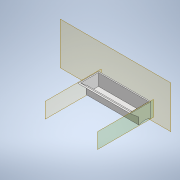
# Autodesk Inventor part: sump
Saved by Autodesk Inventor 2022 (Build 260153000, 153)
## iProperties
Created: 2022-02-25
Part Number: sump
Material: Generic
Document SubType Name: Modeling
Designer: efred
Density: 1 g/cm^3
Appearance: Default
Author: efred
Autodesk Inventor part; units mm, degrees
ref_plane "YZ Plane" through (0, 0, 0) normal (1, 0, 0) x (0, 1, 0)
ref_plane "XZ Plane" through (0, 0, 0) normal (0, 1, 0) x (-1, 0, 0)
ref_plane "XY Plane" through (0, 0, 0) normal (0, 0, 1) x (1, 0, 0)
ref_plane "Work Plane1" through (0, 0, 0) normal (0, 0, 1) x (1, 0, 0)
ref_plane "Work Plane2" through (157.5, -135.5375, 119.9) normal (1, 0, 0) x (0, 0, -1)
ref_plane "Work Plane3" through (404.675, -135.5375, 119.9) normal (-1, 0, 0) x (0, 0, 1)
sketch "Sketch2" plane through (404.675, -135.5375, 119.9) normal (-1, 0, 0) x (0, 0, 1)
  line L0 (-120, -33.125) -> (-120, 33.125) projected
  line L1 (120, -33.125) -> (-120, -33.125) projected
  line L2 (120, 33.125) -> (120, -33.125) projected
  line L3 (-120, 33.125) -> (120, 33.125) projected
  circle A0 centre (7, 26.125) radius 1.95 projected
  circle A1 centre (113, -26.875) radius 1.95 projected
  circle A2 centre (113, 12.125) radius 1.95 projected
  circle A3 centre (99, 26.125) radius 1.95 projected
  circle A4 centre (-55, -26.875) radius 1.95 projected
  line L4 (0.75, 33.125) -> (-62, -20.125) projected
  line L5 (-50.0649, 0.1287) -> (-21.3323, 24.6904) projected
  line L6 (-11.7313, 32.1577) -> (-59.0108, -8.2587) projected
  line L7 (-62, -22.3139) -> (-62, -29.97) projected
  line L8 (-119.9, -33.125) -> (-62.2, -33.125)
  line L9 (-62.2, -33.125) -> (-62.2, 33.125)
  line L10 (-62.2, 33.125) -> (-119.9, 33.125)
  line L11 (-119.9, 33.125) -> (-119.9, -33.125)
  line L12 (-62.2, 33.125) -> (-22.5461, 33.125)
  line L13 (-22.5461, 33.125) -> (-62.2, -0.7727)
  line L14 (-50.1997, 8.8278) -> (-29.9045, 26.1769) projected
  point P0 (-119.9, 135.5375)
  point P1 (-119.9, 33.125)
  point P2 (-119.9, -33.125)
  point P3 (-62.2, -33.125)
  dimension "d2" = 0.1
  dimension "d3" = 0.2
  dimension "d16" = 0.5
  constraints: 12 end point, 3 parallel, 3 point on line, 1 collinear, 1 horizontal, 1 perpendicular
  measures "d2" distance between parallel lines of L0 L11
  measures "d3" distance between parallel lines of L7 L9
  measures "d16" distance between parallel lines of L14 L13
extrude "Extrusion1" add sketch "Sketch2" along normal up to surface (247.175 mm away) contours L11 L3 L9 L1 | L3 L13 L9
shell "Shell1" thickness 5 removed faces 1 at (322.2833, -102.4125, 64.9026)
sketch "Sketch3" plane through (404.675, -135.5375, 119.9) normal (1, 0, 0) x (0, 0, -1)
  line L0 (114.9, -28.125) -> (67.2, -28.125) projected
  line L1 (67.2, -28.125) -> (67.2, 1.531) projected
  line L2 (115, 28.125) -> (115, -28.125) projected
  line L3 (67.2, -23.125) -> (115, -23.125)
  line L4 (115, -23.125) -> (115, -28.125)
  line L5 (115, -28.125) -> (67.2, -28.125)
  line L6 (67.2, -28.125) -> (67.2, -23.125)
  point P0 (119.9, 135.5375)
  point P1 (115, -23.125)
  dimension "d8" = 5
  constraints: 8 end point, 2 parallel, 1 horizontal, 1 perpendicular, 1 point on line
  measures "d8" distance between parallel lines of L0 L3
extrude "Extrusion2" add sketch "Sketch3" against normal up to surface (242.175 mm away)
sketch "Sketch4" plane through (404.675, -135.5375, 119.9) normal (1, 0, 0) x (0, 0, -1)
  line L0 (119.9, -33.125) -> (62.2, -33.125) projected
  arc A0 (114.9, -33.125) -> (67.2, -33.125) centre (91.05, -87.5073) ccw
  point P0 (119.9, 135.5375)
  point P1 (91.05, -28.125)
  point P2 (91.05, -33.125)
  dimension "d12" = 5
  dimension "d13" = 5
  constraints: 3 point on circle, 2 point on line, 1 centre point, 1 midpoint, 1 vertical alignment
  measures "d12" distance of L0.start A0.start
  measures "d13" distance of point (91.05, -33.125) point (91.05, -28.125)
extrude "Extrusion3" cut sketch "Sketch4" against normal through all
body "Solid1"
